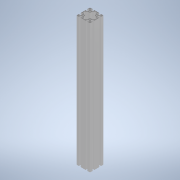
# Autodesk Inventor part: 40-8080-25-CL
Saved by Autodesk Inventor 2021 (Build 250183000, 183)
## iProperties
Category: PARTsolutions
Company: 8020
Part Number: 40-8080-25-CL
Material: Aluminum 6061
Catalog Web Link: www.cadenas.de
Description: 40-8080, 40-8080-Black-T-Slotted Profile - 40 Series
Vendor: 8020
Document SubType Name: Modeling
Designer: partserver
Manufacturer: 8020
Mass: 161.572 g
Surface Area: 286.332 cm^2
Volume: 59.8413 cm^3
Density: 2.7 g/cm^3
Appearance: Aluminum - Flat
PSOL_IDENT_0: {$CADENAS_DATA\23d-libs\8020\metric\profiles\40_series\40_8080.prj},188 {VTYP=3D},{NB=40-8080-25-CL}
PSOL_IDENT_1: ,{LINA=40-8080-25},{NN=40-8080, 40-8080-Black},{DATE=31.07.2020 09:21:33},{GEOMDATE=07.11.2018 21:04
PSOL_IDENT_2: :00},{VERSION=},{LINEID=10},{WBVAR=FIN,LS,L},{WBNUMERIC=L}  {NB=40-8080-25-CL},{LINA=40-8080-25},{KT=
PSOL_IDENT_3: DUMMY},{PN=40-8080-25},{PN1=40-8080},{SERIES=40-8080},{MAT=6105-T5 Aluminum},{FIN=CA},{LS=-CL},{L=25
PSOL_IDENT_4: .00},{LALG=[25:6000/0.05]},{W=6.4280},{MIX=171.6341},{MIY=171.6341},{EA=23.8908},{COLOR=.75,.75,.75}
NB: 40-8080-25-CL
NN: 40-8080, 40-8080-Black
NT: T-Slotted Profile - 40 Series
NBSYN: $PN.$LS.
LINA: 40-8080-25
CATALOG: 80/20
PN: 40-8080-25
SERIES: 40-8080
MAT: 6105-T5 Aluminum
FIN: Clear Anodize
LS: Custom Length
L: 25
W: 6.4280
MIX: 171.6341
MIY: 171.6341
EA: 23.8908
SUPPLIER: 8020
ARTICLENO: 40-8080-25-CL
BOMINFO: 40-8080-25
CREATOR: CADENAS GmbH
Title: 40-8080-25
Author: Cadenas PARTsolutions
Comments: T-Slotted Profile - 40 Series
Autodesk Inventor part; units mm, degrees
sketch "Sketch_1" plane through (0, 0, 0) normal (0, 0, 1) x (1, 0, 0)
  line L0 (-40, 34.365) -> (-40, 5.635)
  arc A0 (-40, 5.635) -> (-38.43, 4.065) centre (-38.43, 5.635) ccw
  line L1 (-38.43, 4.065) -> (-37.25, 4.065)
  arc A1 (-37.25, 4.065) -> (-35.68, 5.635) centre (-37.25, 5.635) ccw
  line L2 (-35.68, 5.635) -> (-35.68, 8.66)
  arc A2 (-34.11, 10.23) -> (-35.68, 8.66) centre (-34.11, 8.66) ccw
  line L3 (-34.11, 10.23) -> (-33.5995, 10.23)
  arc A3 (-33.0621, 10.0074) -> (-33.5995, 10.23) centre (-33.5995, 9.47) ccw
  line L4 (-33.0621, 10.0074) -> (-29.1098, 6.0551)
  arc A4 (-27.685, 2.6153) -> (-29.1098, 6.0551) centre (-32.5496, 2.6153) ccw
  line L5 (-27.685, 2.6153) -> (-27.685, -2.6153)
  arc A5 (-29.1098, -6.0551) -> (-27.685, -2.6153) centre (-32.5496, -2.6153) ccw
  line L6 (-29.1098, -6.0551) -> (-33.0621, -10.0074)
  arc A6 (-33.5995, -10.23) -> (-33.0621, -10.0074) centre (-33.5995, -9.47) ccw
  line L7 (-33.5995, -10.23) -> (-34.11, -10.23)
  arc A7 (-35.68, -8.66) -> (-34.11, -10.23) centre (-34.11, -8.66) ccw
  line L8 (-35.68, -8.66) -> (-35.68, -5.635)
  arc A8 (-35.68, -5.635) -> (-37.25, -4.065) centre (-37.25, -5.635) ccw
  line L9 (-37.25, -4.065) -> (-38.43, -4.065)
  arc A9 (-38.43, -4.065) -> (-40, -5.635) centre (-38.43, -5.635) ccw
  line L10 (-40, -5.635) -> (-40, -16.83)
  arc A10 (-40, -16.83) -> (-36.83, -20) centre (-36.83, -16.83) ccw
  line L11 (-36.83, -20) -> (-25.635, -20)
  arc A11 (-25.635, -20) -> (-24.065, -18.43) centre (-25.635, -18.43) ccw
  line L12 (-24.065, -18.43) -> (-24.065, -17.25)
  arc A12 (-24.065, -17.25) -> (-25.635, -15.68) centre (-25.635, -17.25) ccw
  line L13 (-25.635, -15.68) -> (-28.66, -15.68)
  arc A13 (-30.23, -14.11) -> (-28.66, -15.68) centre (-28.66, -14.11) ccw
  line L14 (-30.23, -14.11) -> (-30.23, -13.5995)
  arc A14 (-30.0074, -13.0621) -> (-30.23, -13.5995) centre (-29.47, -13.5995) ccw
  line L15 (-30.0074, -13.0621) -> (-26.0551, -9.1098)
  arc A15 (-22.6153, -7.685) -> (-26.0551, -9.1098) centre (-22.6153, -12.5496) ccw
  line L16 (-22.6153, -7.685) -> (-17.3847, -7.685)
  arc A16 (-13.9449, -9.1098) -> (-17.3847, -7.685) centre (-17.3847, -12.5496) ccw
  line L17 (-13.9449, -9.1098) -> (-9.9926, -13.0621)
  arc A17 (-9.77, -13.5995) -> (-9.9926, -13.0621) centre (-10.53, -13.5995) ccw
  line L18 (-9.77, -13.5995) -> (-9.77, -14.11)
  arc A18 (-11.34, -15.68) -> (-9.77, -14.11) centre (-11.34, -14.11) ccw
  line L19 (-11.34, -15.68) -> (-14.365, -15.68)
  arc A19 (-14.365, -15.68) -> (-15.935, -17.25) centre (-14.365, -17.25) ccw
  line L20 (-15.935, -17.25) -> (-15.935, -18.43)
  arc A20 (-15.935, -18.43) -> (-14.365, -20) centre (-14.365, -18.43) ccw
  line L21 (-14.365, -20) -> (14.365, -20)
  arc A21 (14.365, -20) -> (15.935, -18.43) centre (14.365, -18.43) ccw
  line L22 (15.935, -18.43) -> (15.935, -17.25)
  arc A22 (15.935, -17.25) -> (14.365, -15.68) centre (14.365, -17.25) ccw
  line L23 (14.365, -15.68) -> (11.34, -15.68)
  arc A23 (9.77, -14.11) -> (11.34, -15.68) centre (11.34, -14.11) ccw
  line L24 (9.77, -14.11) -> (9.77, -13.5995)
  arc A24 (9.9926, -13.0621) -> (9.77, -13.5995) centre (10.53, -13.5995) ccw
  line L25 (9.9926, -13.0621) -> (13.9449, -9.1098)
  arc A25 (17.3847, -7.685) -> (13.9449, -9.1098) centre (17.3847, -12.5496) ccw
  line L26 (17.3847, -7.685) -> (22.6153, -7.685)
  arc A26 (26.0551, -9.1098) -> (22.6153, -7.685) centre (22.6153, -12.5496) ccw
  line L27 (26.0551, -9.1098) -> (30.0074, -13.0621)
  arc A27 (30.23, -13.5995) -> (30.0074, -13.0621) centre (29.47, -13.5995) ccw
  line L28 (30.23, -13.5995) -> (30.23, -14.11)
  arc A28 (28.66, -15.68) -> (30.23, -14.11) centre (28.66, -14.11) ccw
  line L29 (28.66, -15.68) -> (25.635, -15.68)
  arc A29 (25.635, -15.68) -> (24.065, -17.25) centre (25.635, -17.25) ccw
  line L30 (24.065, -17.25) -> (24.065, -18.43)
  arc A30 (24.065, -18.43) -> (25.635, -20) centre (25.635, -18.43) ccw
  line L31 (25.635, -20) -> (36.83, -20)
  arc A31 (36.83, -20) -> (40, -16.83) centre (36.83, -16.83) ccw
  line L32 (40, -16.83) -> (40, -5.635)
  arc A32 (40, -5.635) -> (38.43, -4.065) centre (38.43, -5.635) ccw
  line L33 (38.43, -4.065) -> (37.25, -4.065)
  arc A33 (37.25, -4.065) -> (35.68, -5.635) centre (37.25, -5.635) ccw
  line L34 (35.68, -5.635) -> (35.68, -8.66)
  arc A34 (34.11, -10.23) -> (35.68, -8.66) centre (34.11, -8.66) ccw
  line L35 (34.11, -10.23) -> (33.5995, -10.23)
  arc A35 (33.0621, -10.0074) -> (33.5995, -10.23) centre (33.5995, -9.47) ccw
  line L36 (33.0621, -10.0074) -> (29.1098, -6.0551)
  arc A36 (27.685, -2.6153) -> (29.1098, -6.0551) centre (32.5496, -2.6153) ccw
  line L37 (27.685, -2.6153) -> (27.685, 2.6153)
  arc A37 (29.1098, 6.0551) -> (27.685, 2.6153) centre (32.5496, 2.6153) ccw
  line L38 (29.1098, 6.0551) -> (33.0621, 10.0074)
  arc A38 (33.5995, 10.23) -> (33.0621, 10.0074) centre (33.5995, 9.47) ccw
  line L39 (33.5995, 10.23) -> (34.11, 10.23)
  arc A39 (35.68, 8.66) -> (34.11, 10.23) centre (34.11, 8.66) ccw
  line L40 (35.68, 8.66) -> (35.68, 5.635)
  arc A40 (35.68, 5.635) -> (37.25, 4.065) centre (37.25, 5.635) ccw
  line L41 (37.25, 4.065) -> (38.43, 4.065)
  arc A41 (38.43, 4.065) -> (40, 5.635) centre (38.43, 5.635) ccw
  line L42 (40, 5.635) -> (40, 34.365)
  arc A42 (40, 34.365) -> (38.43, 35.935) centre (38.43, 34.365) ccw
  line L43 (38.43, 35.935) -> (37.25, 35.935)
  arc A43 (37.25, 35.935) -> (35.68, 34.365) centre (37.25, 34.365) ccw
  line L44 (35.68, 34.365) -> (35.68, 31.34)
  arc A44 (34.11, 29.77) -> (35.68, 31.34) centre (34.11, 31.34) ccw
  line L45 (34.11, 29.77) -> (33.5995, 29.77)
  arc A45 (33.0621, 29.9926) -> (33.5995, 29.77) centre (33.5995, 30.53) ccw
  line L46 (33.0621, 29.9926) -> (29.1098, 33.9449)
  arc A46 (27.685, 37.3847) -> (29.1098, 33.9449) centre (32.5496, 37.3847) ccw
  line L47 (27.685, 37.3847) -> (27.685, 42.6153)
  arc A47 (29.1098, 46.0551) -> (27.685, 42.6153) centre (32.5496, 42.6153) ccw
  line L48 (29.1098, 46.0551) -> (33.0621, 50.0074)
  arc A48 (33.5995, 50.23) -> (33.0621, 50.0074) centre (33.5995, 49.47) ccw
  line L49 (33.5995, 50.23) -> (34.11, 50.23)
  arc A49 (35.68, 48.66) -> (34.11, 50.23) centre (34.11, 48.66) ccw
  line L50 (35.68, 48.66) -> (35.68, 45.635)
  arc A50 (35.68, 45.635) -> (37.25, 44.065) centre (37.25, 45.635) ccw
  line L51 (37.25, 44.065) -> (38.43, 44.065)
  arc A51 (38.43, 44.065) -> (40, 45.635) centre (38.43, 45.635) ccw
  line L52 (40, 45.635) -> (40, 56.83)
  arc A52 (40, 56.83) -> (36.83, 60) centre (36.83, 56.83) ccw
  line L53 (36.83, 60) -> (25.635, 60)
  arc A53 (25.635, 60) -> (24.065, 58.43) centre (25.635, 58.43) ccw
  line L54 (24.065, 58.43) -> (24.065, 57.25)
  arc A54 (24.065, 57.25) -> (25.635, 55.68) centre (25.635, 57.25) ccw
  line L55 (25.635, 55.68) -> (28.66, 55.68)
  arc A55 (30.23, 54.11) -> (28.66, 55.68) centre (28.66, 54.11) ccw
  line L56 (30.23, 54.11) -> (30.23, 53.5995)
  arc A56 (30.0074, 53.0621) -> (30.23, 53.5995) centre (29.47, 53.5995) ccw
  line L57 (30.0074, 53.0621) -> (26.0551, 49.1098)
  arc A57 (22.6153, 47.685) -> (26.0551, 49.1098) centre (22.6153, 52.5496) ccw
  line L58 (22.6153, 47.685) -> (17.3847, 47.685)
  arc A58 (13.9449, 49.1098) -> (17.3847, 47.685) centre (17.3847, 52.5496) ccw
  line L59 (13.9449, 49.1098) -> (9.9926, 53.0621)
  arc A59 (9.77, 53.5995) -> (9.9926, 53.0621) centre (10.53, 53.5995) ccw
  line L60 (9.77, 53.5995) -> (9.77, 54.11)
  arc A60 (11.34, 55.68) -> (9.77, 54.11) centre (11.34, 54.11) ccw
  line L61 (11.34, 55.68) -> (14.365, 55.68)
  arc A61 (14.365, 55.68) -> (15.935, 57.25) centre (14.365, 57.25) ccw
  line L62 (15.935, 57.25) -> (15.935, 58.43)
  arc A62 (15.935, 58.43) -> (14.365, 60) centre (14.365, 58.43) ccw
  line L63 (14.365, 60) -> (-14.365, 60)
  arc A63 (-14.365, 60) -> (-15.935, 58.43) centre (-14.365, 58.43) ccw
  line L64 (-15.935, 58.43) -> (-15.935, 57.25)
  arc A64 (-15.935, 57.25) -> (-14.365, 55.68) centre (-14.365, 57.25) ccw
  line L65 (-14.365, 55.68) -> (-11.34, 55.68)
  arc A65 (-9.77, 54.11) -> (-11.34, 55.68) centre (-11.34, 54.11) ccw
  line L66 (-9.77, 54.11) -> (-9.77, 53.5995)
  arc A66 (-9.9926, 53.0621) -> (-9.77, 53.5995) centre (-10.53, 53.5995) ccw
  line L67 (-9.9926, 53.0621) -> (-13.9449, 49.1098)
  arc A67 (-17.3847, 47.685) -> (-13.9449, 49.1098) centre (-17.3847, 52.5496) ccw
  line L68 (-17.3847, 47.685) -> (-22.6153, 47.685)
  arc A68 (-26.0551, 49.1098) -> (-22.6153, 47.685) centre (-22.6153, 52.5496) ccw
  line L69 (-26.0551, 49.1098) -> (-30.0074, 53.0621)
  arc A69 (-30.23, 53.5995) -> (-30.0074, 53.0621) centre (-29.47, 53.5995) ccw
  line L70 (-30.23, 53.5995) -> (-30.23, 54.11)
  arc A70 (-28.66, 55.68) -> (-30.23, 54.11) centre (-28.66, 54.11) ccw
  line L71 (-28.66, 55.68) -> (-25.635, 55.68)
  arc A71 (-25.635, 55.68) -> (-24.065, 57.25) centre (-25.635, 57.25) ccw
  line L72 (-24.065, 57.25) -> (-24.065, 58.43)
  arc A72 (-24.065, 58.43) -> (-25.635, 60) centre (-25.635, 58.43) ccw
  line L73 (-25.635, 60) -> (-36.83, 60)
  arc A73 (-36.83, 60) -> (-40, 56.83) centre (-36.83, 56.83) ccw
  line L74 (-40, 56.83) -> (-40, 45.635)
  arc A74 (-40, 45.635) -> (-38.43, 44.065) centre (-38.43, 45.635) ccw
  line L75 (-38.43, 44.065) -> (-37.25, 44.065)
  arc A75 (-37.25, 44.065) -> (-35.68, 45.635) centre (-37.25, 45.635) ccw
  line L76 (-35.68, 45.635) -> (-35.68, 48.66)
  arc A76 (-34.11, 50.23) -> (-35.68, 48.66) centre (-34.11, 48.66) ccw
  line L77 (-34.11, 50.23) -> (-33.5995, 50.23)
  arc A77 (-33.0621, 50.0074) -> (-33.5995, 50.23) centre (-33.5995, 49.47) ccw
  line L78 (-33.0621, 50.0074) -> (-29.1098, 46.0551)
  arc A78 (-27.685, 42.6153) -> (-29.1098, 46.0551) centre (-32.5496, 42.6153) ccw
  line L79 (-27.685, 42.6153) -> (-27.685, 37.3847)
  arc A79 (-29.1098, 33.9449) -> (-27.685, 37.3847) centre (-32.5496, 37.3847) ccw
  line L80 (-29.1098, 33.9449) -> (-33.0621, 29.9926)
  arc A80 (-33.5995, 29.77) -> (-33.0621, 29.9926) centre (-33.5995, 30.53) ccw
  line L81 (-33.5995, 29.77) -> (-34.11, 29.77)
  arc A81 (-35.68, 31.34) -> (-34.11, 29.77) centre (-34.11, 31.34) ccw
  line L82 (-35.68, 31.34) -> (-35.68, 34.365)
  arc A82 (-35.68, 34.365) -> (-37.25, 35.935) centre (-37.25, 34.365) ccw
  line L83 (-37.25, 35.935) -> (-38.43, 35.935)
  arc A83 (-38.43, 35.935) -> (-40, 34.365) centre (-38.43, 34.365) ccw
  circle A84 centre (20, 0) radius 3.405
  circle A85 centre (20, 40) radius 3.405
  circle A86 centre (-20, 0) radius 3.405
  circle A87 centre (-20, 40) radius 3.405
  arc A88 (-35.68, 15.8732) -> (-34.41, 14.6032) centre (-34.41, 15.8732) ccw
  line L84 (-34.41, 14.6032) -> (-32.0745, 14.6032)
  arc A89 (-31.1765, 14.2312) -> (-32.0745, 14.6032) centre (-32.0745, 13.3332) ccw
  line L85 (-31.1765, 14.2312) -> (-25.5351, 8.5898)
  arc A90 (-25.5351, 8.5898) -> (-22.0953, 7.165) centre (-22.0953, 12.0296) ccw
  line L86 (-22.0953, 7.165) -> (-17.585, 7.165)
  arc A91 (-12.835, 2.415) -> (-17.585, 7.165) centre (-17.585, 2.415) ccw
  line L87 (-12.835, 2.415) -> (-12.835, -2.0953)
  arc A92 (-12.835, -2.0953) -> (-11.4102, -5.5351) centre (-7.9704, -2.0953) ccw
  line L88 (-11.4102, -5.5351) -> (-5.8014, -11.1439)
  arc A93 (-5.4294, -12.0419) -> (-5.8014, -11.1439) centre (-6.6994, -12.0419) ccw
  line L89 (-5.4294, -12.0419) -> (-5.4294, -14.41)
  arc A94 (-5.4294, -14.41) -> (-4.1594, -15.68) centre (-4.1594, -14.41) ccw
  line L90 (-4.1594, -15.68) -> (4.1594, -15.68)
  arc A95 (4.1594, -15.68) -> (5.4294, -14.41) centre (4.1594, -14.41) ccw
  line L91 (5.4294, -14.41) -> (5.4294, -12.0419)
  arc A96 (5.8014, -11.1439) -> (5.4294, -12.0419) centre (6.6994, -12.0419) ccw
  line L92 (5.8014, -11.1439) -> (11.4102, -5.5351)
  arc A97 (11.4102, -5.5351) -> (12.835, -2.0953) centre (7.9704, -2.0953) ccw
  line L93 (12.835, -2.0953) -> (12.835, 2.415)
  arc A98 (17.585, 7.165) -> (12.835, 2.415) centre (17.585, 2.415) ccw
  line L94 (17.585, 7.165) -> (22.0953, 7.165)
  arc A99 (22.0953, 7.165) -> (25.5351, 8.5898) centre (22.0953, 12.0296) ccw
  line L95 (25.5351, 8.5898) -> (31.1765, 14.2312)
  arc A100 (32.0745, 14.6032) -> (31.1765, 14.2312) centre (32.0745, 13.3332) ccw
  line L96 (32.0745, 14.6032) -> (34.41, 14.6032)
  arc A101 (34.41, 14.6032) -> (35.68, 15.8732) centre (34.41, 15.8732) ccw
  line L97 (35.68, 15.8732) -> (35.68, 24.1268)
  arc A102 (35.68, 24.1268) -> (34.41, 25.3968) centre (34.41, 24.1268) ccw
  line L98 (34.41, 25.3968) -> (32.0745, 25.3968)
  arc A103 (31.1765, 25.7688) -> (32.0745, 25.3968) centre (32.0745, 26.6668) ccw
  line L99 (31.1765, 25.7688) -> (25.5351, 31.4102)
  arc A104 (25.5351, 31.4102) -> (22.0953, 32.835) centre (22.0953, 27.9704) ccw
  line L100 (22.0953, 32.835) -> (17.585, 32.835)
  arc A105 (12.835, 37.585) -> (17.585, 32.835) centre (17.585, 37.585) ccw
  line L101 (12.835, 37.585) -> (12.835, 42.0953)
  arc A106 (12.835, 42.0953) -> (11.4102, 45.5351) centre (7.9704, 42.0953) ccw
  line L102 (11.4102, 45.5351) -> (5.8014, 51.1439)
  arc A107 (5.4294, 52.0419) -> (5.8014, 51.1439) centre (6.6994, 52.0419) ccw
  line L103 (5.4294, 52.0419) -> (5.4294, 54.41)
  arc A108 (5.4294, 54.41) -> (4.1594, 55.68) centre (4.1594, 54.41) ccw
  line L104 (4.1594, 55.68) -> (-4.1594, 55.68)
  arc A109 (-4.1594, 55.68) -> (-5.4294, 54.41) centre (-4.1594, 54.41) ccw
  line L105 (-5.4294, 54.41) -> (-5.4294, 52.0419)
  arc A110 (-5.8014, 51.1439) -> (-5.4294, 52.0419) centre (-6.6994, 52.0419) ccw
  line L106 (-5.8014, 51.1439) -> (-11.4102, 45.5351)
  arc A111 (-11.4102, 45.5351) -> (-12.835, 42.0953) centre (-7.9704, 42.0953) ccw
  line L107 (-12.835, 42.0953) -> (-12.835, 37.585)
  arc A112 (-17.585, 32.835) -> (-12.835, 37.585) centre (-17.585, 37.585) ccw
  line L108 (-17.585, 32.835) -> (-22.0953, 32.835)
  arc A113 (-22.0953, 32.835) -> (-25.5351, 31.4102) centre (-22.0953, 27.9704) ccw
  line L109 (-25.5351, 31.4102) -> (-31.1765, 25.7688)
  arc A114 (-32.0745, 25.3968) -> (-31.1765, 25.7688) centre (-32.0745, 26.6668) ccw
  line L110 (-32.0745, 25.3968) -> (-34.41, 25.3968)
  arc A115 (-34.41, 25.3968) -> (-35.68, 24.1268) centre (-34.41, 24.1268) ccw
  line L111 (-35.68, 24.1268) -> (-35.68, 15.8732)
  constraints: 224 end point, 224 point on circle, 116 centre point
extrude "Extrusion1" add sketch "Sketch_1" against normal blind 25
ref_plane "1_XY" through (0, 0, 0) normal (0, 0, 1) x (1, 0, 0)
ref_plane "1_YZ" through (0, 0, 0) normal (1, 0, 0) x (0, 1, 0)
ref_plane "1_ZX" through (0, 0, 0) normal (0, 1, 0) x (0, 0, 1)
ref_plane "to_parts_XY" through (0, 0, -12.5) normal (0, 0, 1) x (1, 0, 0)
ref_plane "to_parts_YZ" through (0, 0, -12.5) normal (1, 0, 0) x (0, 1, 0)
ref_plane "to_parts_ZX" through (0, 0, -12.5) normal (0, 1, 0) x (0, 0, 1)
thicken "Thicken1" operation add thickness 0.4 both sides no extend neighbours yes toward (0, 0, -1) faces at (38.56, 18.6244, -25)
thicken "Thicken2" operation add thickness 736.6 both sides no extend neighbours yes toward (0, 0, -1) faces at (-1.3865, -18.56, -25.4)
ref_plane "Work Plane8" through (-20, 57.25, 0) normal (1, 0, 0) x (0, 0, -1)
body "Solid1"
